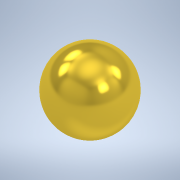
# Autodesk Inventor part: Ball
Saved by Autodesk Inventor 2022.2 (Build 262287030, 287C)
## iProperties
Created: 2022-09-03
Part Number: Ball
Material: Generic
Document SubType Name: Modeling
Designer: fpopa
Density: 1 g/cm^3
Appearance: Metal 2400F Hot
Author: fpopa
Autodesk Inventor part; units mm, degrees
ref_plane "YZ Plane" through (0, 0, 0) normal (1, 0, 0) x (0, 1, 0)
ref_plane "XZ Plane" through (0, 0, 0) normal (0, 1, 0) x (-1, 0, 0)
ref_plane "XY Plane" through (0, 0, 0) normal (0, 0, 1) x (1, 0, 0)
sketch "Sketch1" plane through (0, 0, 0) normal (0, 0, 1) x (1, 0, 0)
  arc A0 (12, 0) -> (-12, 0) centre (0, 0) ccw
  line L0 (-12, 0) -> (12, 0)
  dimension "d0" = 12
  dimension "d1" = 24
  constraints: 2 end point, 2 point on circle, 1 centre point, 1 coincident, 1 horizontal
  measures "d0" radius of A0
  measures "d1" distance of L0.start L0.end
revolve "Revolution1" add sketch "Sketch1" angle 360 about axis through (-12, 0, 0) along (1, 0, 0)
body "Solid1"
